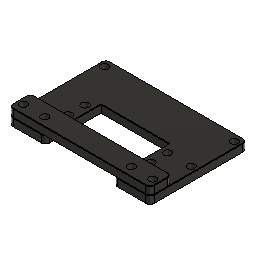
ServoMount (Autodesk Fusion 360 design; units mm, degrees)
Autodesk Fusion 360 part; units mm, degrees
sketch "Sketch1" plane through (0, 0, 0) normal (0, 0, 1) x (1, 0, 0)
  line L0 (-39.3297, 47.5051) -> (-1.8697, 47.5051)
  line L1 (0.6703, 44.9651) -> (0.6703, 30.0451)
  line L2 (-39.3297, 44.9651) -> (-39.3297, 30.0451)
  line L3 (-36.7897, 47.5051) -> (0.6703, 47.5051)
  circle A0 centre (-43.6297, 42.4053) radius 2.159
  circle A1 centre (4.9703, 42.4051) radius 2.159
  circle A2 centre (-43.6297, 32.6053) radius 2.159
  circle A3 centre (4.9703, 32.6051) radius 2.159
  line L4 (-39.3297, 47.5051) -> (-39.3297, 44.9651)
  line L5 (0.6703, 47.5051) -> (0.6703, 44.9651)
  line L6 (-60.9197, 30.0451) -> (-60.9197, 69.4151)
  line L7 (22.2603, 30.0451) -> (22.2603, 69.4151)
  line L8 (19.7203, 71.9551) -> (-58.3797, 71.9551)
  arc A4 (-58.3797, 71.9551) -> (-60.9197, 69.4151) centre (-58.3797, 69.4151) ccw
  arc A5 (22.2603, 69.4151) -> (19.7203, 71.9551) centre (19.7203, 69.4151) ccw
  line L9 (-60.9197, 71.9551) -> (22.2603, 71.9551)
  circle A6 centre (-57.4272, 67.8053) radius 2.159
  circle A7 centre (18.7728, 67.8053) radius 2.159
  circle A8 centre (-57.4272, 19.9053) radius 2.159
  circle A9 centre (-44.7272, 19.9053) radius 2.159
  circle A10 centre (18.7728, 19.9051) radius 2.159
  circle A11 centre (6.0728, 19.9051) radius 2.159
  line L10 (-60.9197, 30.0451) -> (-60.9197, 17.3451)
  line L11 (22.2603, 30.0451) -> (22.2603, 17.3451)
  line L12 (-39.3297, 30.0451) -> (-39.3297, 17.3451)
  line L13 (0.6703, 30.0451) -> (0.6703, 17.3451)
  line L14 (19.7203, 14.8051) -> (3.2103, 14.8051)
  line L15 (-41.8697, 14.8051) -> (-58.3797, 14.8051)
  arc A12 (-60.9197, 17.3451) -> (-58.3797, 14.8051) centre (-58.3797, 17.3451) ccw
  arc A13 (-41.8697, 14.8051) -> (-39.3297, 17.3451) centre (-41.8697, 17.3451) ccw
  arc A14 (0.6703, 17.3451) -> (3.2103, 14.8051) centre (3.2103, 17.3451) ccw
  arc A15 (19.7203, 14.8051) -> (22.2603, 17.3451) centre (19.7203, 17.3451) ccw
  circle A16 centre (-30.1476, 67.8053) radius 2.159
  circle A17 centre (-2.868, 67.8053) radius 2.159
  line L16 (-57.4272, 67.8053) -> (-19.3272, 67.8053)
  circle A18 centre (4.9703, 42.4051) radius 2.159
  line L17 (18.7728, 67.8053) -> (18.7728, 19.9051)
  circle A19 centre (4.9703, 42.4051) radius 2.159
  circle A20 centre (4.9703, 42.4051) radius 2.159
  line L18 (4.9703, 42.4051) -> (4.9703, 71.9551)
  line L19 (4.9703, 42.4051) -> (18.7728, 42.4051)
  circle A21 centre (18.7728, 42.4051) radius 2.159
  line L20 (18.7728, 42.4051) -> (-57.4272, 42.4051)
  point P0 (-54.3297, 57.5051)
  point P1 (-60.9197, 27.5051)
  point P2 (-60.9197, 71.9551)
  point P3 (22.2603, 27.5051)
  point P4 (22.2603, 71.9551)
  point P5 (-60.9197, 14.8051)
  point P6 (22.2603, 14.8051)
  dimension "d11" = 4.318
  dimension "d14" = 4.318
  dimension "d15" = 9.8
  dimension "d16" = 4.318
  dimension "d17" = 9.8
  dimension "d18" = 4.318
  dimension "d49" = 44.45
  dimension "d51" = 44.45
  dimension "d52" = 2.54
  dimension "d54" = 4.318
  dimension "d66" = 4.318
  dimension "d82" = 4.318
  dimension "d84" = 4.318
  dimension "d86" = 4.318
  dimension "d88" = 4.318
  dimension "d89" = 15.24
  dimension "d90" = 15.24
  dimension "d93" = 2.54
  dimension "d108" = 54.5592
  dimension "d109" = 0
  dimension "d110" = 38.1
  dimension "d112" = 4.318
  dimension "d113" = 4.318
  dimension "d114" = 4.318
  dimension "d115" = 4.318
  constraint horizontal L0
  constraint vertical L1
  constraint vertical L2
  constraint horizontal L3
  constraint coincident L0.start L2
  constraint coincident L0 L3.end
  constraint coincident L3.end L1
  constraint coincident P2 L6
  constraint coincident P2 L8
  constraint tangent L6 A4
  constraint tangent L8 A4
  constraint coincident P4 L7
  constraint coincident P4 L8
  constraint tangent L7 A5
  constraint tangent L8 A5
  constraint equal A4 A5
  constraint coincident P3 L7
  constraint coincident P1 L6
  constraint coincident P2 L9.start
  constraint coincident P4 L9.end
  constraint collinear L14 L15
  constraint coincident P5 L10
  constraint coincident P5 L15
  constraint tangent L10 A12
  constraint tangent L15 A12
  constraint tangent L12 A13
  constraint tangent L15 A13
  constraint equal A12 A13
  constraint tangent L13 A14
  constraint tangent L14 A14
  constraint equal A12 A14
  constraint coincident P6 L11
  constraint coincident P6 L14
  constraint tangent L11 A15
  constraint tangent L14 A15
  constraint equal A12 A15
  constraint coincident A6.centre L16.start
  constraint parallel L8 L16
  constraint coincident A7.centre L17.start
  constraint coincident A10.centre L17.end
  constraint parallel L11 L17
  constraint vertical L18
  constraint coincident A1.centre A18.centre
  constraint coincident L8 L18.end
  constraint coincident L17 L19.end
  constraint perpendicular L17 L19
  constraint coincident L19.end A21.centre
  constraint parallel L16 L20
  measures "d11" diameter of A0
  measures "d14" diameter of A1
  measures "d15" distance of A0.centre A2.centre
  measures "d16" diameter of A2
  measures "d17" distance of A1.centre A3.centre
  measures "d18" diameter of A3
  measures "d49" distance of P1 P2
  measures "d51" distance of P3 P4
  measures "d52" radius of A4
  measures "d54" diameter of A6
  measures "d66" diameter of A7
  measures "d82" diameter of A8
  measures "d84" diameter of A9
  measures "d86" diameter of A10
  measures "d88" diameter of A11
  measures "d89" distance of L6.start P5
  measures "d90" distance of L7.start P6
  measures "d93" radius of A12
  measures "d110" distance of A6.centre L16.end
  measures "d112" diameter of A18
  measures "d113" diameter of A19
  measures "d114" diameter of A20
  measures "d115" diameter of A21
sketch "Sketch2" plane through (0, 0, 0) normal (0, 0, 1) x (1, 0, 0)
  line L0 (-41.8969, 27.5037) -> (4.7492, 27.5037)
  line L1 (4.7492, 27.5037) -> (4.7492, 14.7406)
  line L2 (-41.8969, 27.5037) -> (-41.8969, 14.7406)
  line L3 (-41.8969, 14.7406) -> (4.7492, 14.7406)
  constraint horizontal L0
  constraint perpendicular L0 L1
  constraint perpendicular L0 L2
  constraint perpendicular L1 L3
extrude "Extrude4" add sketch "Sketch1" along normal blind 4.7625 contours L0 L1 L2 L3 A1 L4 L5 L6 L8 A4 L9 L10 L12 L15 A12 A13 A18 A19 A20 L18 L20 | L1 A1 L7 L8 A5 L9 L11 L13 L14 A14 A15 A18 A19 A20 L18 L20 | A16 L16 | A16 L16 | A17 makes body 1
sketch "Sketch3" plane through (0, 0, 4.7625) normal (0, 0, 1) x (-1, 0, 0)
  circle A0 centre (-6.0728, -19.9051) radius 2.159
  circle A1 centre (-18.7728, -19.9051) radius 2.159
  circle A2 centre (-4.9703, -32.6051) radius 2.159
  circle A3 centre (57.4272, -19.9053) radius 2.159
  circle A4 centre (44.7272, -19.9053) radius 2.159
  circle A5 centre (43.6297, -42.4053) radius 2.159
  circle A6 centre (57.4272, -67.8053) radius 2.159
  circle A7 centre (-18.7728, -67.8053) radius 2.159
  circle A8 centre (43.6297, -32.6053) radius 2.159
  circle A9 centre (-4.9703, -42.4051) radius 2.159
  line L0 (39.3297, -47.5051) -> (-0.6703, -47.5051)
  line L1 (-0.6703, -47.5051) -> (-0.6703, -17.3451)
  arc A10 (-0.6703, -17.3451) -> (-3.2103, -14.8051) centre (-3.2103, -17.3451) ccw
  line L2 (-3.2103, -14.8051) -> (-19.7203, -14.8051)
  arc A11 (-19.7203, -14.8051) -> (-22.2603, -17.3451) centre (-19.7203, -17.3451) ccw
  line L3 (-22.2603, -17.3451) -> (-22.2603, -69.4151)
  arc A12 (-22.2603, -69.4151) -> (-19.7203, -71.9551) centre (-19.7203, -69.4151) ccw
  line L4 (-19.7203, -71.9551) -> (58.3797, -71.9551)
  arc A13 (58.3797, -71.9551) -> (60.9197, -69.4151) centre (58.3797, -69.4151) ccw
  line L5 (60.9197, -69.4151) -> (60.9197, -17.3451)
  arc A14 (60.9197, -17.3451) -> (58.3797, -14.8051) centre (58.3797, -17.3451) ccw
  line L6 (58.3797, -14.8051) -> (41.8697, -14.8051)
  arc A15 (41.8697, -14.8051) -> (39.3297, -17.3451) centre (41.8697, -17.3451) ccw
  line L7 (39.3297, -17.3451) -> (39.3297, -47.5051)
  line L8 (-0.6703, -27.5033) -> (-19.7213, -27.5033)
  line L9 (-0.6703, -27.5033) -> (58.3797, -27.5033)
  line L10 (60.9197, -24.9633) -> (60.9197, -17.3433)
  line L11 (58.3797, -14.8033) -> (-19.7243, -14.8033)
  line L12 (-22.2643, -17.3443) -> (-22.2613, -24.9643)
  arc A16 (58.3797, -27.5033) -> (60.9197, -24.9633) centre (58.3797, -24.9633) ccw
  arc A17 (-22.2613, -24.9643) -> (-19.7213, -27.5033) centre (-19.7213, -24.9633) ccw
  arc A18 (60.9197, -17.3433) -> (58.3797, -14.8033) centre (58.3797, -17.3433) ccw
  arc A19 (-19.7243, -14.8033) -> (-22.2643, -17.3443) centre (-19.7243, -17.3433) ccw
  circle A20 centre (-18.7728, -42.4051) radius 2.159
  point P0 (60.9197, -27.5033)
  point P1 (60.9197, -14.8033)
  point P2 (-22.2653, -14.8033)
  dimension "d96" = 12.7
  dimension "d97" = 83.185
  dimension "d98" = 2.54
  dimension "d99" = 2.54
  constraint coincident L1 L8.start
  constraint perpendicular L3 L8
  constraint coincident L5 P0
  constraint perpendicular L5 L9
  constraint perpendicular L9 L10
  constraint perpendicular L10 L11
  constraint coincident P0 L9
  constraint coincident P0 L10
  constraint tangent L9 A16
  constraint tangent L10 A16
  constraint tangent L8 A17
  constraint tangent L12 A17
  constraint equal A16 A17
  constraint coincident P1 L10
  constraint coincident P1 L11
  constraint tangent L10 A18
  constraint tangent L11 A18
  constraint coincident P2 L11
  constraint coincident P2 L12
  constraint tangent L11 A19
  constraint tangent L12 A19
  constraint equal A18 A19
  measures "d96" distance of P0 P1
  measures "d97" distance of P1 P2
  measures "d98" radius of A16
  measures "d99" radius of A18
extrude "Extrude5" add sketch "Sketch3" along normal blind 4.7625 separate body contours L1 A10 A15 L7 L9 L11 | L5 A14 L6 A15 L7 L9 L10 L11 A16 A18 | L1 A10 L2 A11 L3 L8 L11 A17 | A11 L3 L12 A19 makes body 2
fillet "Fillet5" radius 0.254 28 edges at (-19.3297, 47.5051, 4.7625) (0.6703, 32.4251, 4.7625) (1.4142, 15.549, 4.7625) (11.4653, 14.8051, 4.7625) (21.5163, 15.549, 4.7625) (22.2603, 43.3801, 4.7625) (21.5163, 71.2111, 4.7625) (-19.3297, 71.9551, 4.7625) (-60.1758, 71.2111, 4.7625) (-60.9197, 43.3801, 4.7625) (-60.1758, 15.549, 4.7625) (-50.1247, 14.8051, 4.7625) (-40.0737, 15.549, 4.7625) (-39.3297, 32.4251, 4.7625) (-19.3297, 47.5051, 0) (0.6703, 32.4251, 0) (1.4142, 15.549, 0) (11.4653, 14.8051, 0) (21.5163, 15.549, 0) (22.2603, 43.3801, 0) (21.5163, 71.2111, 0) (-19.3297, 71.9551, 0) (-60.1758, 71.2111, 0) (-60.9197, 43.3801, 0) (-60.1758, 15.549, 0) (-50.1247, 14.8051, 0) (-40.0737, 15.549, 0) (-39.3297, 32.4251, 0) on bodies 1
fillet "Fillet6" radius 0.254 16 edges at (-60.9197, 21.1533, 9.525) (-60.1758, 15.5473, 9.525) (-19.3277, 14.8033, 9.525) (21.5207, 15.5476, 9.525) (22.2628, 21.1543, 9.525) (21.517, 26.7597, 9.525) (-19.3292, 27.5033, 9.525) (-60.1758, 26.7594, 9.525) (22.2628, 21.1543, 4.7625) (21.517, 26.7597, 4.7625) (-19.3292, 27.5033, 4.7625) (-60.1758, 26.7594, 4.7625) (-60.9197, 21.1533, 4.7625) (-60.1758, 15.5473, 4.7625) (-19.3277, 14.8033, 4.7625) (21.5207, 15.5476, 4.7625) on bodies 2
equation "d94 = ( 3 / 16 ) * 1 in"
equation "d100 = ( 3 / 16 ) * 1 in"
named bodies: "ServoMount", "ServoBar"
